Autodesk Inventor part; units mm, degrees
(part 2 of 2)
sketch "Sketch21" plane through (66.7, 15, 47.7) normal (0, 0, -1) x (-1, 0, 0)
  line L0 (7.228, 0) -> (0, 0) construction
  line L1 (0, 0) -> (0, 16) construction
  line L2 (0, 0) -> (0, 24) construction
  arc A0 (0, 16) -> (0, 24) centre (-8.2956, 20) ccw
  line L3 (0, 24) -> (0, 16)
  point P0 (66.7, -15)
  dimension "d263" = 16
  constraints: 4 end point, 2 point on circle, 1 centre point, 1 collinear, 1 point on line
  measures "d263" distance of L0.end L1.end
extrude "Extrusion19" add sketch "Sketch21" along normal mid plane 3
ref_plane "Work Plane5" through (-10, 15, -57.7) normal (-1, 0, 0) x (0, 0, 1)
ref_plane "Work Plane6" through (66.7, 15, 0) normal (0, 0, -1) x (-1, 0, 0)
mirror "Mirror3" about plane through (-10, 15, -57.7) normal (-1, 0, 0) of "Extrusion19"
mirror "Mirror4" about plane through (66.7, 15, 0) normal (0, 0, -1) of "Extrusion19", "Mirror3"
sketch "Sketch22" plane through (0, 15, 0) normal (0, 1, 0) x (1, 0, 0)
  line L0 (55.857, -25.95) -> (55.857, 25.95) projected
  line L1 (-75.857, 25.95) -> (-75.857, -25.95) projected
  line L2 (30.1507, 0) -> (55.857, 0) construction
  circle A0 centre (43.0038, 0) radius 3.25
  point P0 (0, 0)
  dimension "d268" = 6.5
  constraints: 2 end point, 2 midpoint, 1 centre point
  measures "d268" diameter of A0
extrude "Extrusion20" cut sketch "Sketch22" against normal blind 10
sketch "Sketch23" plane through (0, 15, 0) normal (0, 1, 0) x (1, 0, 0)
  circle A0 centre (43.0038, 0) radius 3.25 projected
  circle A1 centre (43.0038, 0) radius 5.5
  line L0 (40.2024, 6.7598) -> (45.8024, 6.7598)
  line L1 (49.7622, -2.8) -> (49.7622, 2.8)
  line L2 (40.2024, -6.7598) -> (45.8024, -6.7598)
  line L3 (36.2426, 2.8) -> (36.2426, -2.8)
  line L4 (36.2426, 2.8) -> (40.2024, 6.7598)
  line L5 (45.8024, 6.7598) -> (49.7622, 2.8)
  line L6 (49.7622, -2.8) -> (45.8024, -6.7598)
  line L7 (40.2024, -6.7598) -> (36.2426, -2.8)
  line L8 (43.0024, -6.7598) -> (43.0024, 6.7598) construction
  line L9 (-126.685, 0) -> (106.685, 0) construction
  point P0 (0, 0)
  point P1 (39.4683, -3.5355)
  point P2 (43.0038, -5)
  point P3 (38.0024, 2.2881)
  point P4 (46.5394, -3.5355)
  point P5 (48.0024, 2.2945)
  point P6 (47.1595, 3.6028)
  point P7 (43.0038, 5.5)
  point P8 (38.8719, 3.63)
  point P9 (43.0024, 0)
  dimension "d271" = 11
  dimension "d281" = 5.6
  dimension "d282" = 135
  dimension "d283" = 135
  dimension "d284" = 135
  dimension "d285" = 13.5196
  constraints: 18 end point, 7 equal length, 3 midpoint, 2 horizontal, 2 vertical, 1 centre point, 1 coincident, 1 parallel, 1 point on line
  measures "d271" diameter of A1
  measures "d281" distance of L0.end L0.start
  measures "d282" angle of L5 L0
  measures "d283" angle of L1 L5
  measures "d284" angle of L6 L2
  measures "d285" distance between parallel lines of L6 L4
extrude "Extrusion21" cut sketch "Sketch23" against normal blind 6 contours A0 | A1 | L0 L5 L1 L6 L2 L7 L3 L4
sketch "Sketch24" plane through (0, 15, 0) normal (0, 1, 0) x (1, 0, 0)
  circle A0 centre (20, 0) radius 9.5 construction
  line L0 (29.5, 0) -> (38.0038, 0) construction
  circle A1 centre (43.0038, 0) radius 5 construction
  line L1 (33.7519, 0) -> (33.7519, 5) construction
  line L2 (33.7519, 0) -> (33.7519, -5) construction
  arc A2 (34.7519, 5) -> (32.7519, 5) centre (33.7519, 5) ccw
  arc A3 (32.7519, -5) -> (34.7519, -5) centre (33.7519, -5) ccw
  line L3 (32.7519, 5) -> (32.7519, -5)
  line L4 (34.7519, -5) -> (34.7519, 5)
  point P0 (0, 0)
  dimension "d274" = 5
  dimension "d275" = 5
  dimension "d276" = 2
  constraints: 10 end point, 4 point on circle, 3 tangent, 2 centre point, 2 coincident, 2 horizontal alignment, 2 vertical, 1 horizontal, 1 midpoint, 1 parallel, 2 other
  measures "d274" distance of L1.start L1.end
  measures "d275" distance of L1.start L2.end
  measures "d276" diameter of A2
extrude "Extrusion22" cut sketch "Sketch24" against normal through all
mirror "Mirror5" about plane through (-10, 15, -57.7) normal (-1, 0, 0) of "Extrusion21", "Extrusion22"
sketch "Sketch25" plane through (-63.0038, 15, 0) normal (0, 1, 0) x (1, 0, 0)
  circle A0 centre (0, 0) radius 3.25
  point P0 (63.0038, 0)
  constraints: 1 centre point
extrude "Extrusion23" cut sketch "Sketch25" against normal blind 10
body "Solid1"
